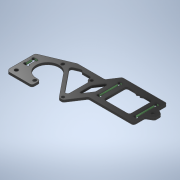
# Autodesk Inventor part: Ankle_side_frame
Saved by Autodesk Inventor 2020 (Build 240168000, 168)
## iProperties
Part Number: Ankle_side_frame
Material: アルミニウム 2014-T4
Document SubType Name: Modeling
Designer: Masato Kubotera
Density: 2.8 g/cm^3
Appearance: 光沢 - 黒
Description: A2017 T2
Mass: 9.74724 g
Surface Area: 49.2982 cm^2
Volume: 3.48116 cm^3
Author: Masato Kubotera
Autodesk Inventor part; units mm, degrees
ref_plane "YZ Plane" through (0, 0, 0) normal (1, 0, 0) x (0, 1, 0)
ref_plane "XZ Plane" through (0, 0, 0) normal (0, 1, 0) x (-1, 0, 0)
ref_plane "XY Plane" through (0, 0, 0) normal (0, 0, 1) x (1, 0, 0)
sketch "スケッチ1" plane through (0, 0, 0) normal (0, 0, 1) x (1, 0, 0)
  line L0 (28, 13.5) -> (1, 13.5) construction
  line L1 (1, 13.5) -> (1, -13.5) construction
  line L2 (1, -13.5) -> (28, -13.5) construction
  line L3 (28, -13.5) -> (28, 13.5) construction
  line L4 (28, 13.5) -> (1, -13.5) construction
  line L5 (1, 13.5) -> (28, -13.5) construction
  circle A0 centre (0, 0) radius 10.5 construction
  arc A1 (0, 16) -> (-12, 10.583) centre (0, 0) ccw construction
  line L6 (1, 0) -> (28, 0) construction
  line L7 (14.5, 13.5) -> (14.5, -13.5) construction
  circle A2 centre (28, 13.5) radius 1.35
  arc A3 (-0.35, 13) -> (2.35, 13) centre (1, 13) ccw
  line L8 (2.35, 13.5) -> (2.35, 13)
  line L9 (-0.35, 13.5) -> (-0.35, 13)
  arc A4 (2.35, 13.5) -> (-0.35, 13.5) centre (1, 13.5) ccw
  line L10 (-12, 10.583) -> (-12, -10.583) construction
  arc A5 (-12, -10.583) -> (0, -16) centre (0, 0) ccw construction
  circle A6 centre (28, -13.5) radius 1.35
  line L11 (-17.5, 5) -> (-14.5, 5) construction
  line L12 (-14.5, 5) -> (-14.5, -5) construction
  line L13 (-14.5, -5) -> (-17.5, -5) construction
  line L14 (-17.5, -5) -> (-17.5, 5) construction
  line L15 (-17.5, 5) -> (-14.5, -5) construction
  line L16 (-14.5, 5) -> (-17.5, -5) construction
  line L17 (-17.525, 5.025) -> (-14.475, 5.025)
  line L18 (-14.475, 5.025) -> (-14.475, 2.925) construction
  line L19 (-14.475, -5.025) -> (-17.525, -5.025)
  line L20 (-17.525, -5.025) -> (-17.525, -2.925) construction
  line L21 (-17.525, 5.025) -> (-14.475, -5.025) construction
  line L22 (-14.475, 5.025) -> (-17.525, -5.025) construction
  arc A7 (-17.525, 5.025) -> (-17.525, 2.925) centre (-17.525, 3.975) ccw
  line L23 (-17.5, 0) -> (-14.5, 0) construction
  line L24 (-16, 5) -> (-16, -5) construction
  arc A8 (-14.475, 2.925) -> (-14.475, 5.025) centre (-14.475, 3.975) ccw
  arc A9 (-17.525, -2.925) -> (-17.525, -5.025) centre (-17.525, -3.975) ccw
  arc A10 (-14.475, -5.025) -> (-14.475, -2.925) centre (-14.475, -3.975) ccw
  line L25 (-17.525, 2.925) -> (-17.525, 5.025) construction
  line L26 (-17.525, -2.925) -> (-17.525, 2.925)
  line L27 (-14.475, -2.925) -> (-14.475, -5.025) construction
  line L28 (-14.475, 2.925) -> (-14.475, -2.925)
  line L29 (-20.5, 8.739) -> (-20.5, -15.7058)
  line L30 (-3.2261, 16) -> (30.4, 16) construction
  circle A11 centre (28, 13.5) radius 2.4 construction
  circle A12 centre (28, -13.5) radius 2.4 construction
  circle A13 centre (83.5, 15.5) radius 1.6
  line L31 (83.5, 12.0359) -> (80.5, 13.7679) construction
  line L32 (80.5, 13.7679) -> (80.5, 17.2321) construction
  line L33 (80.5, 17.2321) -> (83.5, 18.9641) construction
  line L34 (83.5, 18.9641) -> (86.5, 17.2321) construction
  line L35 (86.5, 17.2321) -> (86.5, 13.7679) construction
  line L36 (86.5, 13.7679) -> (83.5, 12.0359) construction
  line L37 (40, 30.4) -> (82.5, 30.4)
  line L38 (82.5, 30.4) -> (82.5, 21.8509)
  line L39 (82.5, 21.8509) -> (88.5, 18.3868)
  line L40 (88.5, 18.3868) -> (88.5, 12.6132)
  line L41 (88.5, 12.6132) -> (82.5, 9.1491)
  line L42 (82.5, 9.1491) -> (82.5, -1.4)
  line L43 (82.5, -1.4) -> (40, -1.4)
  line L44 (30.4, -16) -> (40, -1.4)
  line L45 (40, 30.4) -> (40, -1.4) construction
  line L46 (32, 8.9311) -> (32, -1.125)
  line L47 (33.8356, -1.6744) -> (38.8356, 5.9298)
  line L48 (39, 6.4792) -> (39, 16.4316)
  line L49 (37.1679, 16.9863) -> (32.1679, 9.4858)
  line L50 (-17.5, 10) -> (-14.5, 10) construction
  line L51 (-14.5, -10) -> (-17.5, -10) construction
  line L52 (-17.5, 10) -> (-14.5, -10) construction
  line L53 (-14.5, 10) -> (-17.5, -10) construction
  line L54 (40, 30.4) -> (33.5063, 20.5242)
  line L55 (30.4, 16) -> (30.4, -16) construction
  line L56 (43, 25.4) -> (45, 25.4) construction
  line L57 (45, 25.4) -> (45, 3.6) construction
  line L58 (45, 3.6) -> (43, 3.6) construction
  line L59 (43, 3.6) -> (43, 25.4) construction
  line L60 (43, 25.4) -> (45, 3.6) construction
  line L61 (45, 25.4) -> (43, 3.6) construction
  line L62 (42.975, 25.425) -> (45.025, 25.425)
  line L63 (45.025, 25.425) -> (45.025, 23.325) construction
  line L64 (45.025, 3.575) -> (42.975, 3.575)
  line L65 (42.975, 3.575) -> (42.975, 5.675) construction
  line L66 (42.975, 25.425) -> (45.025, 3.575) construction
  line L67 (45.025, 25.425) -> (42.975, 3.575) construction
  line L68 (44, 25.4) -> (44, 3.6) construction
  line L69 (43, 14.5) -> (45, 14.5) construction
  arc A14 (42.975, 25.425) -> (42.975, 23.325) centre (42.975, 24.375) ccw
  arc A15 (45.025, 23.325) -> (45.025, 25.425) centre (45.025, 24.375) ccw
  arc A16 (42.975, 5.675) -> (42.975, 3.575) centre (42.975, 4.625) ccw
  arc A17 (45.025, 3.575) -> (45.025, 5.675) centre (45.025, 4.625) ccw
  line L70 (45.025, 23.325) -> (45.025, 5.675)
  line L71 (42.975, 5.675) -> (42.975, 23.325)
  line L72 (45.025, 5.675) -> (45.025, 3.575) construction
  line L73 (28, 9.4689) -> (28, -7.0627)
  arc A18 (8.3509, 6.7694) -> (-10.75, 0) centre (0, 0) ccw
  line L74 (8.3509, 6.7694) -> (26.0579, -15.0743)
  arc A19 (26.0579, -15.0743) -> (28, -16) centre (28, -13.5) ccw
  line L75 (7.8297, 12.1764) -> (24.4463, -8.3221)
  line L76 (-20.5, 8.739) -> (7.5369, 20.5242)
  line L77 (-20.5, -15.7058) -> (-18.8868, -18.5)
  line L78 (-14.2679, -16.5) -> (-17.7321, -16.5) construction
  line L79 (-17.7321, -16.5) -> (-19.4641, -13.5) construction
  line L80 (-19.4641, -13.5) -> (-17.7321, -10.5) construction
  line L81 (-17.7321, -10.5) -> (-14.2679, -10.5)
  line L82 (-14.2679, -10.5) -> (-12.5359, -13.5) construction
  line L83 (-12.5359, -13.5) -> (-14.2679, -16.5) construction
  line L84 (3.75, -18.5) -> (-18.8868, -18.5)
  circle A20 centre (-16, -13.5) radius 1.6
  line L85 (28, -16) -> (30.4, -16)
  line L86 (0, -16) -> (30.4, -16) construction
  arc A21 (24.4463, -8.3221) -> (28, -7.0627) centre (26, -7.0627) ccw
  arc A22 (2.35, -13) -> (-0.35, -13) centre (1, -13) ccw
  line L87 (-0.35, -13.5) -> (-0.35, -13)
  arc A23 (-0.35, -13.5) -> (2.35, -13.5) centre (1, -13.5) ccw
  line L88 (2.35, -13.5) -> (2.35, -13)
  arc A24 (-10.75, 0) -> (0, -10.75) centre (0, 0) ccw
  line L89 (0, -10.75) -> (3.75, -10.75)
  line L90 (3.75, -10.75) -> (3.75, -18.5)
  circle A25 centre (1, -13.5) radius 2.75 construction
  line L91 (73.5, 23.4) -> (73.5, 5.6)
  line L92 (71.5, 3.6) -> (51, 3.6)
  line L93 (49, 5.6) -> (49, 23.4)
  arc A26 (51, 25.4) -> (49, 23.4) centre (51, 23.4) ccw
  arc A27 (49, 5.6) -> (51, 3.6) centre (51, 5.6) ccw
  arc A28 (71.5, 3.6) -> (73.5, 5.6) centre (71.5, 5.6) ccw
  line L94 (42.975, 23.325) -> (42.975, 25.425) construction
  line L95 (77.5, 25.4) -> (79.5, 25.4) construction
  line L96 (79.5, 25.4) -> (79.5, 3.6) construction
  line L97 (77.475, 5.675) -> (77.475, 23.325)
  line L98 (78.5, 25.4) -> (78.5, 3.6) construction
  line L99 (79.5, 25.4) -> (77.5, 3.6) construction
  line L100 (77.5, 3.6) -> (77.5, 25.4) construction
  line L101 (77.5, 25.4) -> (79.5, 3.6) construction
  line L102 (79.525, 25.425) -> (77.475, 3.575) construction
  line L103 (77.475, 25.425) -> (79.525, 3.575) construction
  line L104 (79.5, 3.6) -> (77.5, 3.6) construction
  line L105 (79.525, 3.575) -> (77.475, 3.575)
  line L106 (77.475, 3.575) -> (77.475, 5.675) construction
  line L107 (79.525, 23.325) -> (79.525, 5.675)
  line L108 (79.525, 25.425) -> (79.525, 23.325) construction
  line L109 (77.475, 25.425) -> (79.525, 25.425)
  arc A29 (79.525, 3.575) -> (79.525, 5.675) centre (79.525, 4.625) ccw
  line L110 (79.525, 5.675) -> (79.525, 3.575) construction
  arc A30 (77.475, 5.675) -> (77.475, 3.575) centre (77.475, 4.625) ccw
  arc A31 (79.525, 23.325) -> (79.525, 25.425) centre (79.525, 24.375) ccw
  line L111 (77.5, 14.5) -> (79.5, 14.5) construction
  line L112 (77.475, 23.325) -> (77.475, 25.425) construction
  arc A32 (77.475, 25.425) -> (77.475, 23.325) centre (77.475, 24.375) ccw
  arc A33 (38.8356, 5.9298) -> (39, 6.4792) centre (38, 6.4792) ccw
  arc A34 (39, 16.4316) -> (37.1679, 16.9863) centre (38, 16.4316) ccw
  arc A35 (32.1679, 9.4858) -> (32, 8.9311) centre (33, 8.9311) ccw
  arc A36 (32, -1.125) -> (33.8356, -1.6744) centre (33, -1.125) ccw
  line L113 (30.4, 0) -> (40, 14.5) construction
  line L114 (59.0179, 24.534) -> (57.9821, 25.1321)
  line L115 (51, 25.4) -> (56.9821, 25.4)
  arc A37 (62.116, 24.9) -> (60.384, 24.9) centre (61.25, 24.4) ccw
  arc A38 (57.9821, 25.1321) -> (56.9821, 25.4) centre (56.9821, 23.4) ccw
  arc A39 (59.0179, 24.534) -> (60.384, 24.9) centre (59.5179, 25.4) ccw
  line L116 (61.25, 24.4) -> (61.25, 25.4) construction
  line L117 (63.4821, 24.534) -> (64.5179, 25.1321)
  arc A40 (65.5179, 25.4) -> (64.5179, 25.1321) centre (65.5179, 23.4) ccw
  arc A41 (62.116, 24.9) -> (63.4821, 24.534) centre (62.9821, 25.4) ccw
  line L118 (71.5, 25.4) -> (65.5179, 25.4)
  arc A42 (73.5, 23.4) -> (71.5, 25.4) centre (71.5, 23.4) ccw
  line L119 (59.5179, 24.4) -> (62.9821, 24.4) construction
  line L120 (33.5063, 20.5242) -> (7.5369, 20.5242)
  line L121 (8.6084, 15.2796) -> (13.5764, 17.3679)
  arc A43 (8.6084, 15.2796) -> (7.8297, 12.1764) centre (9.3834, 13.4359) ccw
  arc A44 (16.0927, 16.5081) -> (13.5764, 17.3679) centre (14.3514, 15.5242) ccw
  line L122 (16.9633, 16) -> (23.5279, 16)
  arc A45 (16.0927, 16.5081) -> (16.9633, 16) centre (16.9633, 17) ccw
  line L123 (12.7012, 17) -> (15.7012, 17) construction
  line L124 (12.7012, 17) -> (12.7012, 16) construction
  arc A46 (25.5155, 13.7778) -> (26.8889, 11.2605) centre (28, 13.5) ccw
  arc A47 (25.5155, 13.7778) -> (23.5279, 16) centre (23.5279, 14) ccw
  arc A48 (28, 9.4689) -> (26.8889, 11.2605) centre (26, 9.4689) ccw
  point P0 (14.5, 0)
  point P1 (-16, 0)
  point P2 (-16, 0)
  point P3 (32, 9.2339)
  point P4 (32, -4.4659)
  point P5 (39, 6.1799)
  point P6 (39, 19.7346)
  point P7 (44, 14.5)
  point P8 (-16, 0)
  point P9 (73.5, 25.4)
  point P10 (78.5, 14.5)
  point P11 (6.1514, 14.2468)
  point P12 (57.5179, 25.4)
  point P13 (16.294, 16)
  point P14 (28, 16)
  point P15 (28, 11)
  dimension "d0" = 27
  dimension "d1" = 27
  dimension "d2" = 21
  dimension "d6" = 2.7
  dimension "d9" = 0.5
  dimension "d10" = 1.35
  dimension "d11" = 1
  dimension "d12" = 16
  dimension "d13" = 12
  dimension "d14" = 3
  dimension "d16" = 2.5
  dimension "d18" = 0.025
  dimension "d28" = 3
  dimension "d29" = 4.8
  dimension "d53" = 4.8
  dimension "d54" = 10
  dimension "d55" = 0.025
  dimension "d56" = 1.05
  dimension "d80" = 3.2
  dimension "d87" = 2
  dimension "d88" = 2
  dimension "d90" = 2
  dimension "d91" = 6
  dimension "d109" = 5
  dimension "d113" = 1.05
  dimension "d118" = 45
  dimension "d120" = 4
  dimension "d121" = 4
  dimension "d122" = 3
  dimension "d124" = 14.5
  dimension "d135" = 17
  dimension "d136" = 20
  dimension "d141" = 0.25
  dimension "d143" = 3
  dimension "d144" = 6
  dimension "d145" = 2
  dimension "d146" = 2
  dimension "d148" = 0.5
  dimension "d149" = 3.2
  dimension "d151" = 2
  dimension "d153" = 5.5
  dimension "d154" = 2
  dimension "d158" = 21.8
  dimension "d159" = 0.025
  dimension "d160" = 5
  dimension "d171" = 2
  dimension "d173" = 4
  dimension "d175" = 0.025
  dimension "d178" = 34.5
  dimension "d183" = 4
  dimension "d184" = 1
  dimension "d185" = 3
  dimension "d186" = 1
  dimension "d187" = 1
  dimension "d188" = 5
  dimension "d191" = 1
  dimension "d199" = 2
  dimension "d200" = 1
  dimension "d201" = 1
  dimension "d202" = 30
  dimension "d203" = 2
  dimension "d204" = 2
  dimension "d205" = 1
  dimension "d206" = 1
  constraints: 252 end point, 89 point on circle, 49 centre point, 45 tangent, 38 parallel, 36 midpoint, 36 point on line, 28 symmetric about line, 16 perpendicular, 15 horizontal, 12 coincident, 7 vertical, 5 collinear, 5 equal radius, 1 concentric, 84 other
  measures "d0" distance of L2.end L1.end
  measures "d1" distance of L1.end L0.end
  measures "d2" diameter of A0
  measures "d6" diameter of A2
  measures "d9" distance of A3.centre L0.end
  measures "d10" radius of A4
  measures "d11" distance of point (0, 0) L6.start
  measures "d12" radius of A1
  measures "d13" distance from line of L10 A0.centre
  measures "d14" distance of L12.end L13.end
  measures "d16" distance between parallel lines of L10 L12
  measures "d18" distance between parallel lines of L17 L11
  measures "d28" distance between parallel lines of L29 L14
  measures "d29" diameter of A11
  measures "d53" diameter of A12
  measures "d54" distance between parallel lines of L13 L11
  measures "d55" distance between parallel lines of L14 L25
  measures "d56" radius of A7
  measures "d80" diameter of A13
  measures "d87" distance between parallel lines of L40 L35
  measures "d88" distance between parallel lines of L39 L34
  measures "d90" distance between parallel lines of L41 L36
  measures "d91" distance between parallel lines of L36 L33
  measures "d109" distance between parallel lines of L11 L50
  measures "d113" radius of A14
  measures "d118" distance from line of L57 point (0, 0)
  measures "d120" distance between parallel lines of L73 L46
  measures "d121" distance between parallel lines of L59 L48
  measures "d122" distance between parallel lines of L45 L59
  measures "d124" distance between parallel lines of L6 L69
  measures "d135" distance from line of point (-16, 0) L1
  measures "d136" distance between parallel lines of L51 L50
  measures "d141" radial gap between concentric circles of A18 A0
  measures "d143" distance between parallel lines of L74 L75
  measures "d144" distance between parallel lines of L78 L81
  measures "d145" distance between parallel lines of L77 L79
  measures "d146" distance between parallel lines of L84 L78
  measures "d148" distance between parallel lines of L81 L51
  measures "d149" diameter of A20
  measures "d151" radius of A21
  measures "d153" diameter of A25
  measures "d154" distance of L57.end L58.end
  measures "d158" distance between parallel lines of L58 L56
  measures "d159" distance between parallel lines of L56 L62
  measures "d160" distance between parallel lines of L43 L58
  measures "d171" radius of A26
  measures "d173" distance between parallel lines of L57 L93
  measures "d175" distance between parallel lines of L59 L94
  measures "d178" distance of L56.start L95.start
  measures "d183" distance between parallel lines of L91 L100
  measures "d184" distance from line of A13.centre L111
  measures "d185" distance between parallel lines of L38 L96
  measures "d186" distance between parallel lines of L96 L32
  measures "d187" radius of A33
  measures "d188" distance between parallel lines of L44 L47
  measures "d191" radius of A37
  measures "d199" radius of A38
  measures "d200" radius of A39
  measures "d201" distance from line of L119 L116.end
  measures "d202" angle of L114 L115
  measures "d203" radius of A43
  measures "d204" radius of A44
  measures "d205" radius of A45
  measures "d206" distance of L123.start L124.end
extrude "押し出し1" add sketch "スケッチ1" along normal blind 2
fillet "フィレット1" radius 2 16 edges at (-20.5, 8.739, 1) (-20.5, -15.7058, 1) (-18.8868, -18.5, 1) (40, 30.4, 1) (82.5, 30.4, 1) (82.5, 21.8509, 1) (88.5, 18.3868, 1) (88.5, 12.6132, 1) (82.5, 9.1491, 1) (82.5, -1.4, 1) (40, -1.4, 1) (30.4, -16, 1) (3.75, -18.5, 1) (3.75, -10.75, 1) (33.5063, 20.5242, 1) (7.5369, 20.5242, 1)
equation "\"d10\" = 0.5 * d6"
